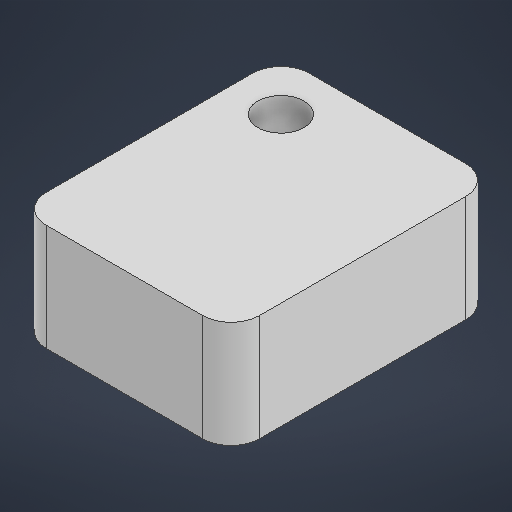
# Autodesk Inventor part: Maintaining_piece_IMU
Saved by Autodesk Inventor 2026.1 (Build 301233000, 233)
## iProperties
Created: 2025-06-10
Part Number: Maintaining_piece_IMU
Material: Générique
Document SubType Name: Modeling
Designer: ewenm
Density: 1 g/cm^3
Appearance: Par défaut
Author: ewenm
Autodesk Inventor part; units mm, degrees
ref_plane "YZ Plane" through (0, 0, 0) normal (1, 0, 0) x (0, 1, 0)
ref_plane "XZ Plane" through (0, 0, 0) normal (0, 1, 0) x (-1, 0, 0)
ref_plane "XY Plane" through (0, 0, 0) normal (0, 0, 1) x (1, 0, 0)
sketch "Esquisse1" plane through (0, 0, 0) normal (0, 1, 0) x (-1, 0, 0)
  line L0 (6.9167, 9.25) -> (-8.0833, 9.25)
  line L1 (-8.0833, 9.25) -> (-8.0833, -9.25)
  line L2 (-8.0833, -9.25) -> (6.9167, -9.25)
  line L3 (6.9167, -9.25) -> (6.9167, 9.25)
  circle A0 centre (3.4167, -5.75) radius 1.625
  point P0 (0, 0)
  dimension "d0" = 9.25
  dimension "d1" = 9.25
  dimension "d2" = 15
  dimension "d3" = 3.25
  dimension "d4" = 3.5
  dimension "d5" = 3.5
  constraints: 8 end point, 2 parallel, 1 centre point, 1 horizontal, 1 perpendicular
  measures "d0" distance from line of point (0, 0) L0
  measures "d1" distance from line of L2 point (0, 0)
  measures "d2" distance between parallel lines of L3 L1
  measures "d3" diameter of A0
  measures "d4" distance from line of L3 A0.centre
  measures "d5" distance from line of L2 A0.centre
extrude "Extrusion1" add sketch "Esquisse1" along normal blind 7.5
fillet "Congé1" radius 2 4 edges at (8.0833, 3.75, 9.25) (8.0833, 3.75, -9.25) (-6.9167, 3.75, -9.25) (-6.9167, 3.75, 9.25)
